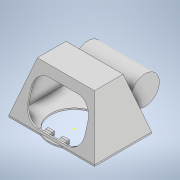
# Autodesk Inventor part: кольцо башни
Saved by Autodesk Inventor 2020.1 (Build 241239000, 239)
## iProperties
Created: 2022-03-20
Part Number: кольцо башни
Material: Типовые
Document SubType Name: Modeling
Designer: User
Density: 1 g/cm^3
Appearance: По умолчанию
Author: User
Autodesk Inventor part; units mm, degrees
ref_plane "YZ Plane" through (0, 0, 0) normal (1, 0, 0) x (0, 1, 0)
ref_plane "XZ Plane" through (0, 0, 0) normal (0, 1, 0) x (-1, 0, 0)
ref_plane "XY Plane" through (0, 0, 0) normal (0, 0, 1) x (1, 0, 0)
sketch "Эскиз1" plane through (0, 0, 0) normal (0, 1, 0) x (-1, 0, 0)
  circle A0 centre (0, 0) radius 35
  circle A1 centre (0, 0) radius 33
  line L0 (15, 31.6228) -> (-15, 31.6228)
  line L1 (15, 31.6228) -> (15, 21.6228)
  line L2 (15, 21.6228) -> (-15, 21.6228)
  line L3 (-15, 21.6228) -> (-15, 31.6228)
  line L4 (60, 31.6228) -> (-60, 31.6228)
  line L5 (-60, 31.6228) -> (-60, -48.3772)
  line L6 (-60, -48.3772) -> (60, -48.3772)
  line L7 (60, -48.3772) -> (60, 31.6228)
  line L8 (0, 35) -> (0, -35)
  point P0 (0, -33)
  point P1 (15, 29.3939)
  point P2 (-15, 29.3939)
  point P3 (-9.434, 31.6228)
  point P4 (9.434, 31.6228)
  dimension "d0" = 70
  dimension "d1" = 2
  dimension "d4" = 30
  dimension "d5" = 10
  dimension "d19" = 0
  dimension "d20" = 120
  dimension "d21" = 80
  constraints: 18 end point, 5 perpendicular, 4 point on circle, 2 coincident, 2 horizontal, 2 parallel, 1 centre point, 4 other
  measures "d0" diameter of A0
  measures "d1" distance of L8.end point (0, -33)
  measures "d4" distance of L0.start L0.end
  measures "d5" distance of L2.end L0.end
  measures "d19" vertical distance of L0.start L4.start
  measures "d20" distance of L5.end L6.end
  measures "d21" distance of L6.end L4.start
extrude "Выдавливание1" add sketch "Эскиз1" along normal blind 2 contours A0 L8 A1 L1 | A0 L4 L7 L6 L5 | L0 A1 L8 A0 | L1 A1 L0 | A0 L3 A1 L8 | L8 A1 L0 A0 | L0 L8 A1 | L0 A1 L3 | L8 L0 A1
sketch "Эскиз2" plane through (0, 0, 0) normal (0, -1, 0) x (1, 0, 0)
  arc A0 (15, 31.6228) -> (-15, 31.6228) centre (0, 0) ccw projected
  line L0 (15, 31.6228) -> (-15, 31.6228)
  line L1 (-15, 31.6228) -> (-15, 21.6228)
  line L2 (-15, 21.6228) -> (15, 21.6228)
  line L3 (15, 21.6228) -> (15, 31.6228)
  arc A1 (-15, 31.6228) -> (0, 35) centre (0, 0) ccw
  dimension "d6" = 30
  dimension "d7" = 10
  constraints: 8 end point, 6 point on circle, 2 perpendicular, 1 centre point, 1 concentric, 1 horizontal, 1 vertical
  measures "d6" distance of L0.start L0.end
  measures "d7" distance of L2.end L0.start
extrude "Выдавливание2" add sketch "Эскиз2" against normal blind 10 contours L3 L2 L1 L0
sketch "Эскиз3" plane through (15, 0, 29.3939) normal (1, 0, 0) x (0, 0, -1)
  circle A0 centre (2.7711, 6) radius 2
  line L0 (7.7711, 10) -> (-2.2289, 10) projected
  point P0 (29.3939, 0)
  point P1 (2.7711, 10)
  dimension "d10" = 4
  dimension "d11" = 0
  dimension "d12" = 4
  constraints: 1 centre point, 1 midpoint
  measures "d10" diameter of A0
  measures "d11" horizontal distance of point (2.771, 10) A0.centre
  measures "d12" distance from line of L0 A0.centre
extrude "Выдавливание3" cut sketch "Эскиз3" against normal blind 100
fillet "Сопряжение1" radius 2 2 edges at (0, 10, 21.6228) (0, 10, 31.6228)
sketch "Эскиз4" plane through (0, 10, 0) normal (0, 1, 0) x (1, 0, 0)
  line L0 (-15, -21.6228) -> (15, -21.6228) projected
  line L1 (0, -21.6228) -> (0, -31.6228)
  line L2 (-15, -31.6228) -> (15, -31.6228) projected
  line L3 (6, -21.6228) -> (-6, -21.6228)
  line L4 (-6, -21.6228) -> (-6, -31.6228)
  line L5 (-6, -31.6228) -> (6, -31.6228)
  line L6 (6, -31.6228) -> (6, -21.6228)
  point P0 (0, 0)
  dimension "d16" = 12
  constraints: 10 end point, 2 midpoint, 2 parallel, 2 point on line, 1 horizontal, 1 perpendicular, 1 other
  measures "d16" distance of L3.start L3.end
extrude "Выдавливание4" cut sketch "Эскиз4" against normal blind 10
sketch "Эскиз5" plane through (60, 0, -48.3772) normal (0, 0, -1) x (-1, 0, 0)
  line L0 (60, 0) -> (60, 63.6764)
  line L1 (20, 72) -> (100, 72)
  line L2 (0, 2) -> (120, 2) projected
  line L3 (0, 2) -> (20, 72)
  line L4 (100, 72) -> (120, 2)
  line L5 (2.08, 2) -> (21.5086, 70)
  line L6 (21.5086, 70) -> (98.4914, 70)
  line L7 (98.4914, 70) -> (117.92, 2)
  dimension "d22" = 70
  dimension "d23" = 80
  dimension "d24" = 2
  dimension "d25" = 2
  dimension "d26" = 2
  constraints: 14 end point, 3 parallel, 2 point on line, 1 horizontal, 1 vertical, 1 other
  measures "d22" distance from line of L2 L1.start
  measures "d23" distance of L1.start L1.end
  measures "d24" distance from line of L1 L6.end
  measures "d25" distance from line of L4 L6.end
  measures "d26" distance from line of L3 L5.end
extrude "Выдавливание5" add sketch "Эскиз5" against normal mid plane 160 contours L1 L4 L2 L7 L6 L5 L3
sketch "Эскиз6" plane through (60, 0, 31.6228) normal (1, 0, 0) x (0, 0, -1)
  line L0 (0, 2) -> (80, 2) projected
  line L1 (0, 72) -> (160, 72) projected
  line L2 (0, 70) -> (160, 70) projected
  line L3 (2.2289, 2) -> (0, 2) projected
  line L4 (0, 2) -> (20, 72)
  line L5 (20, 72) -> (60, 72)
  line L6 (60, 72) -> (80, 2)
  line L7 (40, 70) -> (40, 2)
  line L8 (0, 0) -> (80, 0) projected
  line L9 (170.7435, -15.7415) -> (-33.7928, -15.7415)
  line L10 (-33.7928, -15.7415) -> (-33.7928, 98.2589)
  line L11 (-33.7928, 98.2589) -> (170.7435, 98.2589)
  line L12 (170.7435, 98.2589) -> (170.7435, -15.7415)
  line L13 (0, 2) -> (-3.3772, 2) projected
  line L14 (80, 0) -> (80, 2) projected
  line L15 (-3.3772, 2) -> (80, 2)
  line L16 (80, 2) -> (80, 0)
  line L17 (80, 0) -> (-3.3772, 0)
  line L18 (-3.3772, 0) -> (-3.3772, 2)
  point P0 (31.6228, 0)
  point P1 (40, 72)
  dimension "d29" = 40
  constraints: 24 end point, 4 parallel, 4 point on line, 3 perpendicular, 2 horizontal, 1 midpoint, 1 other
  measures "d29" distance of L5.end L4.end
extrude "Выдавливание6" cut sketch "Эскиз6" against normal blind 1000
sketch "Эскиз8" plane through (60, 0, 31.6228) normal (1, 0, 0) x (0, 0, -1)
  line L0 (80, 2) -> (60.5714, 70) projected
  line L1 (80, 2) -> (60.5714, 70)
  line L2 (60.5714, 70) -> (58.5714, 70)
  line L3 (19.4286, 70) -> (60.5714, 70) projected
  line L4 (58.5714, 70) -> (78, 2)
  line L5 (80, 2) -> (0, 2) projected
  line L6 (78, 2) -> (80, 2)
  line L7 (19.4286, 70) -> (0, 2) projected
  line L8 (19.4286, 70) -> (0, 2)
  line L9 (0, 2) -> (2, 2)
  line L10 (80, 2) -> (0, 2) projected
  line L11 (2, 2) -> (21.4286, 70)
  line L12 (21.4286, 70) -> (19.4286, 70)
  point P0 (31.6228, 0)
  point P1 (2, 2)
  dimension "d32" = 2
  dimension "d42" = 2
  constraints: 16 end point, 4 point on line, 2 collinear, 2 parallel
  measures "d32" distance of L0.end L2.end
  measures "d42" distance of L5.end L9.end
extrude "Выдавливание7" add sketch "Эскиз8" against normal blind 120 contours L5 L4 L2 L0 | L5 L7 L3 L11
sketch "Эскиз9" plane through (60, 0, -48.3772) normal (0, 0, -1) x (-1, 0, 0)
  line L0 (0, 0) -> (0, 2) projected
  line L1 (0, 2) -> (19.5856, 70.5494)
  line L2 (21.5086, 70) -> (2.08, 2) projected
  line L3 (19.5856, 70.5494) -> (-29.2522, 76.299)
  line L4 (-29.2522, 76.299) -> (0, 2)
  line L5 (100.5714, 70) -> (120, 2) projected
  line L6 (117.92, 2) -> (120, 2) projected
  line L7 (100.5714, 70) -> (120, 2)
  line L8 (120, 2) -> (219.6358, 73.4242)
  line L9 (100.5714, 70) -> (120, 70) projected
  line L10 (219.6358, 73.4242) -> (100.5714, 70)
  point P0 (60, 0)
  constraints: 12 end point, 1 parallel
extrude "Выдавливание8" cut sketch "Эскиз9" against normal blind 100
sketch "Эскиз10" plane through (0, 0, 0) normal (1, 0, 0) x (0, 1, 0)
  circle A0 centre (37.228, -59.1124) radius 20
  line L0 (2, -48.3772) -> (72, -28.3772) projected
  circle A1 centre (20.1206, -45.2799) radius 2
  circle A2 centre (44.4455, -38.33) radius 2
  point P0 (0, 0)
  point P1 (43.7893, -40.2193)
  point P2 (43.896, -36.4069)
  point P3 (31.7336, -39.8819)
  point P4 (19.5712, -43.3569)
  point P5 (21.6758, -46.5374)
  dimension "d37" = 40
  dimension "d40" = 4
  dimension "d41" = 4
  constraints: 5 tangent, 3 centre point
  measures "d37" diameter of A0
  measures "d40" diameter of A1
  measures "d41" diameter of A2
extrude "Выдавливание9" add sketch "Эскиз10" along normal mid plane 80 contours A0 | A0 L0 A2 | A1 L0 A0
sketch "Эскиз11" plane through (15, 0, 31.6228) normal (0, 0, 1) x (1, 0, 0)
  line L0 (-55, 72) -> (25, 72) projected
  line L1 (-15, 72) -> (-15, 0)
  circle A0 centre (-35, 25) radius 20
  line L2 (-75, 0) -> (-30, 0) projected
  circle A1 centre (5, 25) radius 20
  line L3 (0, 0) -> (45, 0) projected
  line L4 (-35, 45) -> (5, 45)
  line L5 (5, 5) -> (-35, 5)
  circle A2 centre (-35, 40.0469) radius 20
  circle A3 centre (5, 40) radius 20.0469
  line L6 (-35, 60.0469) -> (5, 60.0469)
  line L7 (-55, 40.0469) -> (-55, 25)
  line L8 (-55, 43.896) -> (-55, 19.5712) projected
  line L9 (25, 19.5712) -> (25, 43.896) projected
  line L10 (25, 25) -> (25, 38.6301)
  point P0 (-15, 25)
  point P1 (25, 41.3699)
  point P2 (-53.531, 32.5234)
  point P3 (23.5657, 32.4374)
  point P4 (-15.623, 45)
  point P5 (-14.4133, 45)
  dimension "d43" = 40
  dimension "d44" = 20
  dimension "d45" = 25
  dimension "d46" = 40
  dimension "d47" = 20
  dimension "d48" = 25
  dimension "d51" = 15
  constraints: 12 end point, 10 point on circle, 5 tangent, 4 centre point, 3 point on line, 1 midpoint, 1 vertical
  measures "d43" diameter of A0
  measures "d44" distance from line of L1 A0.centre
  measures "d45" distance from line of L2 A0.centre
  measures "d46" diameter of A1
  measures "d47" distance from line of L1 A1.centre
  measures "d48" distance from line of L3 A1.centre
  measures "d51" distance of A1.centre A3.centre
extrude "Выдавливание10" cut sketch "Эскиз11" against normal blind 40 contours L6 A3 L4 L1 | L1 L4 A2 L6 | L4 A3 L1 | L1 A3 A2 L4 | A2 L4 A0 | A3 L9 A1 L4 | A3 L4 A1 L1 | L1 A2 A3 | A2 A3 A0 L4 | A2 A0 L7 | A2 A3 | L1 A3 A2 | A0 A2 | A1 A3 | A2 A0 | L9 A1 A3 | A3 A1 L1 | L1 A0 A2 A3 | A1 A3 | A0 L1 L5 | A1 L5 L1
sketch "Эскиз12" plane through (0, 0, 0) normal (1, 0, 0) x (0, 1, 0)
  point P0 (0, 0)
